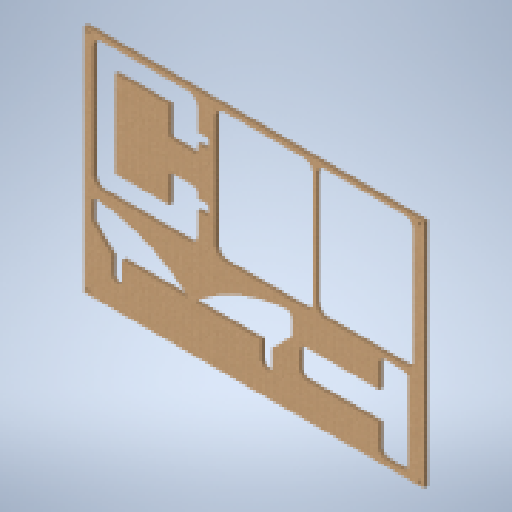
# Autodesk Inventor part: MarcoRompecabezas
Saved by Autodesk Inventor 2023.1 (Build 271208000, 208)
## iProperties
Created: 2022-11-14
Part Number: MarcoRompecabezas
Material: MDF Medium Density Fiberboard
Document SubType Name: Modeling
Designer: Daniel Peña
Density: 0.8 g/cm^3
Appearance: Cardboard - Corrugated
Author: Daniel Peña
Autodesk Inventor part; units mm, degrees
ref_plane "YZ Plane" through (0, 0, 0) normal (1, 0, 0) x (0, 1, 0)
ref_plane "XZ Plane" through (0, 0, 0) normal (0, 1, 0) x (-1, 0, 0)
ref_plane "XY Plane" through (0, 0, 0) normal (0, 0, 1) x (1, 0, 0)
sketch "Sketch1" plane through (0, 0, 0) normal (0, 0, 1) x (1, 0, 0)
  line L0 (-235, -160) -> (-235, 160)
  line L1 (-235, 160) -> (235, 160)
  line L2 (235, 160) -> (235, -160)
  line L3 (235, -160) -> (-235, -160)
  arc A0 (-193.5353, -119.9347) -> (-186.5353, -119.9347) centre (-190.0353, -119.9347) ccw
  line L4 (-197.5353, -97.0737) -> (-197.5353, -119.9347)
  line L5 (-225.0353, -69.5737) -> (-197.5353, -97.0737)
  line L6 (-225.0353, -47.4347) -> (-225.0353, -69.5737)
  arc A1 (-217.5353, -39.9347) -> (-225.0353, -47.4347) centre (-217.5353, -47.4347) ccw
  arc A2 (-90.0353, -94.9347) -> (-217.5353, -39.9347) centre (-235.2895, -256.3762) ccw
  line L7 (-182.5353, -94.9347) -> (-90.0353, -94.9347)
  line L8 (-182.5353, -119.9347) -> (-182.5353, -94.9347)
  arc A3 (-197.5353, -119.9347) -> (-182.5353, -119.9347) centre (-190.0353, -119.9347) ccw
  circle A4 centre (37.1874, -55.0313) radius 3.5
  line L9 (13.6874, -95.0313) -> (13.6874, -120.0313)
  arc A5 (20.6874, -95.0313) -> (13.6874, -95.0313) centre (17.1874, -95.0313) ccw
  line L10 (20.6874, -120.0313) -> (20.6874, -95.0313)
  arc A6 (13.6874, -120.0313) -> (20.6874, -120.0313) centre (17.1874, -120.0313) ccw
  line L11 (24.6874, -97.1703) -> (24.6874, -120.0313)
  line L12 (52.1874, -69.6703) -> (24.6874, -97.1703)
  line L13 (52.1874, -47.5313) -> (52.1874, -69.6703)
  arc A7 (52.1874, -47.5313) -> (44.6874, -40.0313) centre (44.6874, -47.5313) ccw
  arc A8 (44.6874, -40.0313) -> (-82.8126, -95.0313) centre (62.4415, -256.4728) ccw
  line L14 (9.6874, -95.0313) -> (-82.8126, -95.0313)
  line L15 (9.6874, -120.0313) -> (9.6874, -95.0313)
  arc A9 (9.6874, -120.0313) -> (24.6874, -120.0313) centre (17.1874, -120.0313) ccw
  circle A10 centre (66.2275, -11.4924) radius 3.5
  circle A11 centre (-38.7725, 138.5076) radius 3.5
  circle A12 centre (66.2275, 138.5076) radius 3.5
  circle A13 centre (-38.7725, -11.4924) radius 3.5
  line L16 (-23.7725, 13.5076) -> (-23.7725, 113.5076)
  line L17 (51.2275, 13.5076) -> (-23.7725, 13.5076)
  line L18 (51.2275, 113.5076) -> (51.2275, 13.5076)
  line L19 (-23.7725, 113.5076) -> (51.2275, 113.5076)
  arc A14 (-53.7725, -14.4924) -> (-41.7725, -26.4924) centre (-41.7725, -14.4924) ccw
  line L20 (-53.7725, 141.5076) -> (-53.7725, -14.4924)
  arc A15 (-41.7725, 153.5076) -> (-53.7725, 141.5076) centre (-41.7725, 141.5076) ccw
  line L21 (69.2275, 153.5076) -> (-41.7725, 153.5076)
  arc A16 (81.2275, 141.5076) -> (69.2275, 153.5076) centre (69.2275, 141.5076) ccw
  line L22 (81.2275, -14.4924) -> (81.2275, 141.5076)
  arc A17 (69.2275, -26.4924) -> (81.2275, -14.4924) centre (69.2275, -14.4924) ccw
  line L23 (-41.7725, -26.4924) -> (69.2275, -26.4924)
  circle A18 centre (205.99, -10.3277) radius 3.5
  circle A19 centre (100.99, 139.6723) radius 3.5
  circle A20 centre (205.99, 139.6723) radius 3.5
  circle A21 centre (100.99, -10.3277) radius 3.5
  line L24 (115.99, 14.6723) -> (115.99, 114.6723)
  line L25 (190.99, 14.6723) -> (115.99, 14.6723)
  line L26 (190.99, 114.6723) -> (190.99, 14.6723)
  line L27 (115.99, 114.6723) -> (190.99, 114.6723)
  arc A22 (85.99, -13.3277) -> (97.99, -25.3277) centre (97.99, -13.3277) ccw
  line L28 (85.99, 142.6723) -> (85.99, -13.3277)
  arc A23 (97.99, 154.6723) -> (85.99, 142.6723) centre (97.99, 142.6723) ccw
  line L29 (208.99, 154.6723) -> (97.99, 154.6723)
  arc A24 (220.99, 142.6723) -> (208.99, 154.6723) centre (208.99, 142.6723) ccw
  line L30 (220.99, -13.3277) -> (220.99, 142.6723)
  arc A25 (208.99, -25.3277) -> (220.99, -13.3277) centre (208.99, -13.3277) ccw
  line L31 (97.99, -25.3277) -> (208.99, -25.3277)
  circle A26 centre (-103.2457, -11.4392) radius 3.5
  circle A27 centre (-208.2457, 138.5608) radius 3.5
  circle A28 centre (-208.2457, -11.4392) radius 3.5
  circle A29 centre (-103.2457, 138.5608) radius 3.5
  circle A30 centre (-70.7457, 103.5608) radius 3.5
  circle A31 centre (-70.7457, 23.5608) radius 3.5
  arc A32 (-118.2457, 87.5608) -> (-114.2457, 83.5608) centre (-114.2457, 87.5608) ccw
  line L32 (-118.2457, 123.5608) -> (-118.2457, 87.5608)
  line L33 (-193.2457, 123.5608) -> (-118.2457, 123.5608)
  line L34 (-193.2457, 3.5608) -> (-193.2457, 123.5608)
  line L35 (-118.2457, 3.5608) -> (-193.2457, 3.5608)
  line L36 (-118.2457, 39.5608) -> (-118.2457, 3.5608)
  arc A33 (-114.2457, 43.5608) -> (-118.2457, 39.5608) centre (-114.2457, 39.5608) ccw
  line L37 (-82.2457, 43.5608) -> (-114.2457, 43.5608)
  arc A34 (-78.2457, 39.5608) -> (-82.2457, 43.5608) centre (-82.2457, 39.5608) ccw
  line L38 (-78.2457, 31.0608) -> (-78.2457, 39.5608)
  line L39 (-67.2457, 31.0608) -> (-78.2457, 31.0608)
  arc A35 (-63.2457, 27.0608) -> (-67.2457, 31.0608) centre (-67.2457, 27.0608) ccw
  line L40 (-63.2457, 20.0608) -> (-63.2457, 27.0608)
  arc A36 (-67.2457, 16.0608) -> (-63.2457, 20.0608) centre (-67.2457, 20.0608) ccw
  line L41 (-78.2457, 16.0608) -> (-67.2457, 16.0608)
  line L42 (-78.2457, -14.4392) -> (-78.2457, 16.0608)
  arc A37 (-90.2457, -26.4392) -> (-78.2457, -14.4392) centre (-90.2457, -14.4392) ccw
  line L43 (-211.2457, -26.4392) -> (-90.2457, -26.4392)
  arc A38 (-223.2457, -14.4392) -> (-211.2457, -26.4392) centre (-211.2457, -14.4392) ccw
  line L44 (-223.2457, 141.5608) -> (-223.2457, -14.4392)
  arc A39 (-211.2457, 153.5608) -> (-223.2457, 141.5608) centre (-211.2457, 141.5608) ccw
  line L45 (-90.2457, 153.5608) -> (-211.2457, 153.5608)
  circle A40 centre (-210.0353, -54.9347) radius 3.5
  line L46 (-78.2457, 111.0608) -> (-78.2457, 141.5608)
  line L47 (-67.2457, 111.0608) -> (-78.2457, 111.0608)
  arc A41 (-63.2457, 107.0608) -> (-67.2457, 111.0608) centre (-67.2457, 107.0608) ccw
  line L48 (-63.2457, 100.0608) -> (-63.2457, 107.0608)
  arc A42 (-67.2457, 96.0608) -> (-63.2457, 100.0608) centre (-67.2457, 100.0608) ccw
  line L49 (-78.2457, 96.0608) -> (-67.2457, 96.0608)
  line L50 (-78.2457, 87.5608) -> (-78.2457, 96.0608)
  arc A43 (-82.2457, 83.5608) -> (-78.2457, 87.5608) centre (-82.2457, 87.5608) ccw
  line L51 (-114.2457, 83.5608) -> (-82.2457, 83.5608)
  circle A44 centre (70.7997, -92.5277) radius 3.5
  arc A45 (213.2997, -40.5277) -> (205.2997, -32.5277) centre (205.2997, -40.5277) ccw
  line L52 (213.2997, -144.5277) -> (213.2997, -40.5277)
  arc A46 (205.2997, -152.5277) -> (213.2997, -144.5277) centre (205.2997, -144.5277) ccw
  arc A47 (-78.2457, 141.5608) -> (-90.2457, 153.5608) centre (-90.2457, 141.5608) ccw
  arc A48 (173.2997, -144.5277) -> (181.2997, -152.5277) centre (181.2997, -144.5277) ccw
  line L53 (173.2997, -112.5277) -> (173.2997, -144.5277)
  line L54 (71.2997, -112.5277) -> (173.2997, -112.5277)
  arc A49 (63.2997, -104.5277) -> (71.2997, -112.5277) centre (71.2997, -104.5277) ccw
  line L55 (63.2997, -80.5277) -> (63.2997, -104.5277)
  arc A50 (71.2997, -72.5277) -> (63.2997, -80.5277) centre (71.2997, -80.5277) ccw
  line L56 (173.2997, -72.5277) -> (71.2997, -72.5277)
  line L57 (173.2997, -40.5277) -> (173.2997, -72.5277)
  arc A51 (181.2997, -32.5277) -> (173.2997, -40.5277) centre (181.2997, -40.5277) ccw
  line L58 (205.2997, -32.5277) -> (181.2997, -32.5277)
  line L59 (-186.5353, -94.9347) -> (-186.5353, -119.9347)
  arc A52 (-186.5353, -94.9347) -> (-193.5353, -94.9347) centre (-190.0353, -94.9347) ccw
  line L60 (-193.5353, -119.9347) -> (-193.5353, -94.9347)
  line L61 (181.2997, -152.5277) -> (205.2997, -152.5277)
  point P0 (0, 0)
  point P1 (-235, -160)
  dimension "d12" = 6.4392
  constraints: 124 end point, 72 point on circle, 53 centre point, 1 other
  measures "d12" distance between parallel lines of L1 L45
extrude "Extrusion2" add sketch "Sketch1" along normal blind 3 contours L0 L1 L2 L3
sketch "Sketch2" plane through (0, 0, 3) normal (0, 0, 1) x (1, 0, 0)
  line L0 (-235, 160) -> (-235, -160) projected
  line L1 (235, 160) -> (-235, 160) projected
  line L2 (-235, -160) -> (235, -160) projected
  line L3 (235, -160) -> (235, 160) projected
  point P0 (0, 0)
  point P1 (-230, -155)
  point P2 (230, -155)
  point P3 (230, 155)
  point P4 (-230, 155)
  dimension "d4" = 5
  dimension "d5" = 5
  dimension "d6" = 5
  dimension "d7" = 5
  dimension "d8" = 5
  dimension "d9" = 5
  dimension "d10" = 5
  dimension "d11" = 5
  measures "d4" distance from line of L0 point (-230, 155)
  measures "d5" distance from line of L1 point (-230, 155)
  measures "d6" distance from line of L2 point (-230, -155)
  measures "d7" distance from line of point (-230, -155) L0
  measures "d8" distance from line of L2 point (230, -155)
  measures "d9" distance from line of L3 point (230, -155)
  measures "d10" distance from line of L3 point (230, 155)
  measures "d11" distance from line of L1 point (230, 155)
hole "Hole1" at (-230, -155, 3) at (230, -155, 3) at (230, 155, 3) at (-230, 155, 3) direction (0, 0, -1) diameter 5 end through all
equation "\"d4\" = d9"
equation "\"d5\" = d9"
equation "\"d6\" = d9"
equation "\"d7\" = d9"
equation "\"d8\" = d9"
equation "\"d10\" = d9"
equation "\"d11\" = d9"
body "Solid2"
